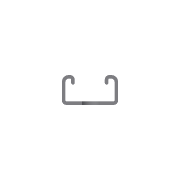
# Autodesk Inventor part: Kevin'sCustomUnistrut
Saved by Autodesk Inventor 2015 (Build 190159000, 159)
## iProperties
Created: 2013-01-12
Part Number: Kevin'sCustomUnistrut
Material: Generic
Document SubType Name: Modeling
Designer: Peter Sloane
Density: 1 g/cm^3
Appearance: Default
Author: Peter Sloane
Autodesk Inventor part; units mm, degrees
ref_plane "YZ Plane" through (0, 0, 0) normal (1, 0, 0) x (0, 1, 0)
ref_plane "XZ Plane" through (0, 0, 0) normal (0, 1, 0) x (-1, 0, 0)
ref_plane "XY Plane" through (0, 0, 0) normal (0, 0, 1) x (1, 0, 0)
sketch "Sketch1" plane through (0, 0, 0) normal (0, 0, 1) x (1, 0, 0)
  arc A0 (38.1698, 2.667) -> (38.9636, 3.4607) centre (38.1698, 3.4607) ccw
  line L0 (38.1698, 2.667) -> (3.4607, 2.667)
  arc A1 (2.667, 3.4607) -> (3.4607, 2.667) centre (3.4607, 3.4607) ccw
  line L1 (2.667, 3.4607) -> (2.667, 17.1767)
  arc A2 (5.0482, 19.558) -> (2.667, 17.1767) centre (5.0482, 17.1767) ccw
  line L2 (5.0482, 19.558) -> (6.4198, 19.558)
  arc A3 (7.2136, 18.7642) -> (6.4198, 19.558) centre (6.4198, 18.7642) ccw
  line L3 (7.2136, 18.7642) -> (7.2136, 16.4211)
  arc A4 (7.2136, 16.4211) -> (9.8806, 16.4211) centre (8.5471, 16.4211) ccw
  line L4 (9.8806, 16.4211) -> (9.8806, 18.7642)
  arc A5 (9.8806, 18.7642) -> (6.4198, 22.225) centre (6.4198, 18.7642) ccw
  line L5 (6.4198, 22.225) -> (5.0482, 22.225)
  arc A6 (5.0482, 22.225) -> (0, 17.1767) centre (5.0482, 17.1767) ccw
  line L6 (0, 17.1767) -> (0, 3.4607)
  arc A7 (0, 3.4607) -> (3.4607, 0) centre (3.4607, 3.4607) ccw
  line L7 (3.4607, 0) -> (38.1698, 0)
  arc A8 (38.1698, 0) -> (41.6306, 3.4607) centre (38.1698, 3.4607) ccw
  line L8 (41.6306, 3.4607) -> (41.6306, 17.1767)
  arc A9 (41.6306, 17.1767) -> (36.5823, 22.225) centre (36.5823, 17.1767) ccw
  line L9 (36.5823, 22.225) -> (35.5664, 22.225)
  arc A10 (35.5664, 22.225) -> (32.1056, 18.7642) centre (35.5664, 18.7642) ccw
  line L10 (32.1056, 18.7642) -> (32.1056, 16.4211)
  arc A11 (32.1056, 16.4211) -> (34.7726, 16.4211) centre (33.4391, 16.4211) ccw
  line L11 (34.7726, 16.4211) -> (34.7726, 18.7642)
  arc A12 (35.5664, 19.558) -> (34.7726, 18.7642) centre (35.5664, 18.7642) ccw
  line L12 (35.5664, 19.558) -> (36.5824, 19.558)
  arc A13 (38.9636, 17.1767) -> (36.5824, 19.558) centre (36.5823, 17.1767) ccw
  line L13 (38.9636, 17.1767) -> (38.9636, 3.4607)
  line L14 (3.4607, 0) -> (0, 0) construction
  line L15 (0, 0) -> (0, 3.4607) construction
  dimension "d0" = 3.4607
  dimension "d1" = 0.7937
  dimension "d2" = 5.0483
  dimension "d3" = 90
  dimension "d4" = 90
  dimension "d5" = 90
  dimension "d6" = 90
  dimension "d7" = 6.858
  dimension "d8" = 31.75
  dimension "d9" = 38.9636
  dimension "d10" = 22.225
  dimension "d11" = 22.225
  dimension "d12" = 19.558
  dimension "d13" = 5.8039
  dimension "d14" = 5.8039
  constraints: 32 end point, 28 point on circle, 28 tangent, 14 centre point, 8 parallel, 6 concentric, 4 equal radius, 2 perpendicular, 1 coincident, 1 vertical
  measures "d0" radius of A8
  measures "d1" radius of A0
  measures "d2" radius of A9
  measures "d3" angle of L9 L8
  measures "d4" angle of L12 L8
  measures "d5" angle of L8 L7
  measures "d6" angle of L9 L6
  measures "d7" distance between parallel lines of L11 L8
  measures "d8" distance between parallel lines of L4 L8
  measures "d9" distance between parallel lines of L1 L8
  measures "d10" distance between parallel lines of L5 L14
  measures "d11" distance from line of point (0, 0) L9
  measures "d12" distance from line of point (0, 0) L12
  measures "d13" distance from line of L11.start L9
  measures "d14" distance from line of L4.start L9
extrude "Extrusion1" add sketch "Sketch1" along normal blind 1828.8
sketch "Sketch13" plane through (3.4607, 2.667, 0) normal (0, 1, 0) x (1, 0, 0)
  line L0 (16.783, -1806.5496) -> (16.7322, -1806.5496)
  line L1 (9.2392, -1799.0566) -> (9.2392, -1785.4676)
  line L2 (16.7322, -1777.9746) -> (16.783, -1777.9746)
  line L3 (24.276, -1785.4676) -> (24.276, -1799.0566)
  line L4 (34.7091, -1828.8) -> (0, -1828.8) projected
  line L5 (32.1056, 0) -> (32.1056, -1828.8) projected
  line L6 (2.9591, 0) -> (2.9591, -1828.8) projected
  arc A0 (16.7322, -1777.9746) -> (9.2392, -1785.4676) centre (16.7322, -1785.4676) ccw
  arc A1 (24.276, -1785.4676) -> (16.783, -1777.9746) centre (16.783, -1785.4676) ccw
  arc A2 (9.2392, -1799.0566) -> (16.7322, -1806.5496) centre (16.7322, -1799.0566) ccw
  arc A3 (16.783, -1806.5496) -> (24.276, -1799.0566) centre (16.783, -1799.0566) ccw
  point P0 (-3.4607, 0)
  point P1 (38.1698, -1828.8)
  point P2 (-3.4608, -1828.8)
  dimension "d146" = 22.2504
  dimension "d147" = 28.575
  dimension "d150" = 13.8938
  dimension "d151" = 12.7
  dimension "d152" = 7.493
  dimension "d153" = 7.493
  dimension "d154" = 7.493
  dimension "d155" = 7.493
  constraints: 8 end point, 8 point on circle, 8 tangent, 4 centre point, 2 parallel, 1 horizontal, 1 perpendicular
  measures "d146" distance between parallel lines of L4 L0
  measures "d147" distance between parallel lines of L2 L0
  measures "d150" distance from line of point (38.17, -1828.8) L3
  measures "d151" distance from line of point (-3.461, -1828.8) L1
  measures "d152" radius of A0
  measures "d153" radius of A1
  measures "d154" radius of A2
  measures "d155" radius of A3
extrude "Extrusion14" cut sketch "Sketch13" against normal blind 25.4
pattern_linear "Rectangular Pattern2" count 36 spacing 51.5112 along (0, 0, -1) of "Extrusion14"
body "Solid1"
